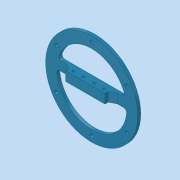
# Autodesk Inventor part: rearServoAttachmentPlate
Saved by Autodesk Inventor 2017 (Build 210142000, 142)
## iProperties
Created: 2016-10-29
Part Number: rearServoAttachmentPlate
Material: ABS Plastic
Document SubType Name: Modeling
Designer: techn
Density: 1.06 g/cm^3
Appearance: Sky Blue Dark
Mass: 24.8742 g
Surface Area: 153.691 cm^2
Volume: 23.4662 cm^3
Author: techn
Autodesk Inventor part; units mm, degrees
ref_plane "YZ Plane" through (0, 0, 0) normal (1, 0, 0) x (0, 1, 0)
ref_plane "XZ Plane" through (0, 0, 0) normal (0, 1, 0) x (-1, 0, 0)
ref_plane "XY Plane" through (0, 0, 0) normal (0, 0, 1) x (1, 0, 0)
sketch "Sketch1" plane through (0, 0, 0) normal (0, 0, 1) x (1, 0, 0)
  circle A0 centre (0, 0) radius 47.625
  dimension "d0" = 95.25
  constraints: 1 centre point, 1 coincident
  measures "d0" diameter of A0
extrude "Extrusion1" add sketch "Sketch1" along normal blind 3.175
sketch "Sketch3" plane through (0, 0, 3.175) normal (0, 0, 1) x (1, 0, 0)
  line L0 (1.27, 9.525) -> (20.32, 9.525)
  line L1 (20.32, 9.525) -> (20.32, 0)
  line L2 (20.32, 0) -> (1.27, 0)
  line L3 (1.27, 0) -> (1.27, 9.525)
  line L4 (0, 0) -> (0, -11.0035)
  line L5 (-1.27, 9.525) -> (-20.32, 9.525)
  line L6 (-20.32, 9.525) -> (-20.32, 0)
  line L7 (-20.32, 0) -> (-1.27, 0)
  line L8 (-1.27, 0) -> (-1.27, 9.525)
  dimension "d11" = 19.05
  dimension "d12" = 9.525
  dimension "d13" = 1.27
  dimension "d14" = 0
  constraints: 18 end point, 4 symmetric about line, 2 parallel, 1 horizontal, 1 perpendicular, 1 vertical
  measures "d11" distance of L1.end L2.end
  measures "d12" distance of L0.end L1.end
  measures "d13" distance from line of L3 L4.start
  measures "d14" distance from line of L2 L4.start
extrude "Extrusion3" add sketch "Sketch3" along normal blind 6.604
sketch "Sketch4" plane through (1.27, 9.525, 3.175) normal (0, 1, 0) x (1, 0, 0)
  circle A0 centre (4.445, -2.794) radius 1.397
  line L0 (19.05, -6.604) -> (0, -6.604) projected
  circle A1 centre (14.605, -2.794) radius 1.397
  line L1 (9.525, -6.604) -> (9.525, -7.9119)
  line L2 (-1.27, 3.175) -> (-1.27, 8.3959)
  circle A2 centre (-6.985, -2.794) radius 1.397
  circle A3 centre (-17.145, -2.794) radius 1.397
  dimension "d17" = 2.794
  dimension "d18" = 3.81
  dimension "d19" = 2.794
  dimension "d20" = 3.81
  dimension "d21" = 10.16
  dimension "d22" = 5.08
  constraints: 4 centre point, 4 end point, 2 symmetric about line, 2 vertical, 1 midpoint, 2 other
  measures "d17" diameter of A0
  measures "d18" distance from line of L0 A0.centre
  measures "d19" diameter of A1
  measures "d20" distance from line of L0 A1.centre
  measures "d21" distance of A1.centre A0.centre
  measures "d22" distance from line of L1 A0.centre
extrude "Extrusion4" cut sketch "Sketch4" against normal through all
sketch "Sketch5" plane through (0, 0, 3.175) normal (0, 0, 1) x (1, 0, 0)
  circle A0 centre (20.795, 25.8191) radius 3.175
  line L0 (0, 0) -> (0, 16.9345)
  circle A1 centre (-20.795, 25.8191) radius 3.175
  dimension "d25" = 6.35
  dimension "d26" = 20.795
  dimension "d27" = 25.8191
  constraints: 2 centre point, 2 end point, 1 symmetric about line, 1 vertical, 1 other
  measures "d25" diameter of A0
  measures "d26" horizontal distance of A0.centre L0.start
  measures "d27" vertical distance of A0.centre L0.start
extrude "Extrusion5" cut sketch "Sketch5" against normal blind 25.4
sketch "Sketch6" plane through (0, 0, 3.175) normal (0, 0, 1) x (1, 0, 0)
  line L0 (0, 0) -> (0, 41.91)
  circle A0 centre (0, 41.91) radius 1.8415
  circle A1 centre (-36.2951, 20.955) radius 1.8415
  circle A2 centre (-36.2951, -20.955) radius 1.8415
  circle A3 centre (0, -41.91) radius 1.8415
  circle A4 centre (36.2951, -20.955) radius 1.8415
  circle A5 centre (36.2951, 20.955) radius 1.8415
  dimension "d30" = 41.91
  dimension "d31" = 3.683
  dimension "d34" = 360
  constraints: 6 centre point, 2 end point, 1 coincident, 1 vertical, 13 other
  measures "d30" distance of L0.start L0.end
  measures "d31" diameter of A0
extrude "Extrusion6" cut sketch "Sketch6" against normal blind 25.4
sketch "Sketch9" plane through (0, 0, 3.175) normal (0, 0, 1) x (1, 0, 0)
  circle A0 centre (0, 0) radius 36.322
  line L0 (-1.27, 9.525) -> (-20.32, 9.525) projected
  line L1 (-20.32, 9.525) -> (-20.32, 0) projected
  line L2 (-20.32, 0) -> (-1.27, 0) projected
  line L3 (-1.27, 0) -> (-1.27, 9.525) projected
  line L4 (20.32, 9.525) -> (1.27, 9.525) projected
  line L5 (1.27, 9.525) -> (1.27, 0) projected
  line L6 (1.27, 0) -> (20.32, 0) projected
  line L7 (20.32, 0) -> (20.32, 9.525) projected
  line L8 (-20.32, 0) -> (-20.32, 9.525) projected
  line L9 (-20.32, 9.525) -> (-35.0508, 9.525)
  line L10 (-20.32, 0) -> (-36.322, 0)
  line L11 (-1.27, 9.525) -> (-1.27, 0) projected
  line L12 (1.27, 9.525) -> (1.27, 0) projected
  line L13 (-1.27, 9.525) -> (1.27, 9.525)
  line L14 (-1.27, 0) -> (1.27, 0)
  line L15 (20.32, 0) -> (36.322, 0)
  line L16 (20.32, 9.525) -> (35.0508, 9.525)
  point P0 (-28.956, -21.928)
  point P1 (-20.701, -29.8455)
  point P2 (28.956, -21.928)
  constraints: 12 end point, 3 horizontal, 3 perpendicular, 1 coincident, 9 other
extrude "Extrusion9" cut sketch "Sketch9" against normal through all contours A0 L10 L2 L14 L6 L15 | L16 L4 L13 L0 L9 A0
sketch "Sketch10" plane through (-1.27, 9.525, 3.175) normal (0, 1, 0) x (1, 0, 0)
  line L0 (0, 0) -> (0, -6.604) projected
  line L1 (2.54, 0) -> (2.54, -6.604) projected
  line L2 (0, -6.604) -> (2.54, -6.604)
  line L3 (2.54, -6.604) -> (2.54, 0)
  line L4 (2.54, 0) -> (0, 0)
  line L5 (0, 0) -> (0, -6.604)
  point P0 (1.27, 3.175)
  constraints: 8 end point, 2 parallel, 1 horizontal, 1 perpendicular
extrude "Extrusion10" add sketch "Sketch10" against normal up to surface (9.525 mm away)
chamfer "Chamfer1" distance 6.35 distance2 3.175 1 edges at (20.32, 4.7625, 3.175) measured on face at (-30.5643, 3.175, 3.175)
chamfer "Chamfer2" distance 6.35 distance2 3.175 1 edges at (-20.32, 4.7625, 3.175) measured on face at (-30.5643, 3.175, 3.175)
fillet "Fillet3" radius 3.175 4 edges at (-35.0508, 9.525, 1.5875) (-36.322, 0, 1.5875) (35.0508, 9.525, 1.5875) (36.322, 0, 1.5875)
body "Solid1"
